Autodesk Inventor part; units mm, degrees
(part 5 of 6)
  line L1795 (9.94, -14.5874) -> (9.724, -14.8873) construction
  line L1796 (9.724, -14.8873) -> (9.508, -15.1933) construction
  line L1797 (9.508, -15.1933) -> (9.2861, -15.4933) construction
  line L1798 (9.2861, -15.4933) -> (8.986, -15.8833)
  line L1799 (8.986, -15.8833) -> (8.8241, -16.0813)
  spline S547 degree 3 poles (8.8241, -16.0813) (8.8061, -16.1053) (8.6861, -16.2073) (8.6921, -16.2433) knots 58 58 58 58 59 59 59 59
  line L1800 (8.8241, -16.0813) -> (8.8061, -16.1053) construction
  line L1801 (8.8061, -16.1053) -> (8.6861, -16.2073) construction
  line L1802 (8.6861, -16.2073) -> (8.6921, -16.2433) construction
  spline S548 degree 3 poles (8.6921, -16.2433) (8.6981, -16.2553) (8.794, -16.1713) (8.8, -16.1653) knots 59 59 59 59 60 60 60 60
  line L1803 (8.6921, -16.2433) -> (8.6981, -16.2553) construction
  line L1804 (8.6981, -16.2553) -> (8.794, -16.1713) construction
  line L1805 (8.794, -16.1713) -> (8.8, -16.1653) construction
  spline S549 degree 3 poles (8.8, -16.1653) (8.728, -16.2433) (8.6321, -16.3513) (8.524, -16.3753) knots 60 60 60 60 61 61 61 61
  line L1806 (8.8, -16.1653) -> (8.728, -16.2433) construction
  line L1807 (8.728, -16.2433) -> (8.6321, -16.3513) construction
  line L1808 (8.6321, -16.3513) -> (8.524, -16.3753) construction
  spline S550 degree 3 poles (8.524, -16.3753) (8.4821, -16.3333) (8.4821, -16.2673) (8.4821, -16.2073) (8.4821, -15.9613) (8.5721, -15.7033) (8.6381, -15.4693) knots 61 61 61 61 62 62 62 63 63 63 63
  line L1809 (8.524, -16.3753) -> (8.4821, -16.3333) construction
  line L1810 (8.4821, -16.3333) -> (8.4821, -16.2673) construction
  line L1811 (8.4821, -16.2673) -> (8.4821, -16.2073) construction
  line L1812 (8.4821, -16.2073) -> (8.4821, -15.9613) construction
  line L1813 (8.4821, -15.9613) -> (8.5721, -15.7033) construction
  line L1814 (8.5721, -15.7033) -> (8.6381, -15.4693) construction
  spline S551 degree 3 poles (8.6381, -15.4693) (8.788, -14.9773) (8.932, -14.4854) (9.112, -14.0054) knots 63 63 63 63 64 64 64 64
  line L1815 (8.6381, -15.4693) -> (8.788, -14.9773) construction
  line L1816 (8.788, -14.9773) -> (8.932, -14.4854) construction
  line L1817 (8.932, -14.4854) -> (9.112, -14.0054) construction
  spline S552 degree 3 poles (9.112, -14.0054) (9.202, -13.7594) (9.304, -13.5194) (9.406, -13.2854) knots 64 64 64 64 65 65 65 65
  line L1818 (9.112, -14.0054) -> (9.202, -13.7594) construction
  line L1819 (9.202, -13.7594) -> (9.304, -13.5194) construction
  line L1820 (9.304, -13.5194) -> (9.406, -13.2854) construction
  spline S553 degree 3 poles (9.406, -13.2854) (9.454, -13.1654) (9.508, -13.0454) (9.562, -12.9254) knots 65 65 65 65 66 66 66 66
  line L1821 (9.406, -13.2854) -> (9.454, -13.1654) construction
  line L1822 (9.454, -13.1654) -> (9.508, -13.0454) construction
  line L1823 (9.508, -13.0454) -> (9.562, -12.9254) construction
  spline S554 degree 3 poles (9.562, -12.9254) (9.604, -12.8414) (9.664, -12.6314) (9.748, -12.6014) knots 66 66 66 66 67 67 67 67
  line L1824 (9.562, -12.9254) -> (9.604, -12.8414) construction
  line L1825 (9.604, -12.8414) -> (9.664, -12.6314) construction
  line L1826 (9.664, -12.6314) -> (9.748, -12.6014) construction
  spline S555 degree 3 poles (9.748, -12.6014) (9.784, -12.5834) (9.844, -12.5954) (9.886, -12.5834) knots 67 67 67 67 68 68 68 68
  line L1827 (9.748, -12.6014) -> (9.784, -12.5834) construction
  line L1828 (9.784, -12.5834) -> (9.844, -12.5954) construction
  line L1829 (9.844, -12.5954) -> (9.886, -12.5834) construction
  spline S556 degree 3 poles (9.886, -12.5834) (9.916, -12.5714) (9.904, -12.5534) (9.934, -12.5474) knots 68 68 68 68 69 69 69 69
  line L1830 (9.886, -12.5834) -> (9.916, -12.5714) construction
  line L1831 (9.916, -12.5714) -> (9.904, -12.5534) construction
  line L1832 (9.904, -12.5534) -> (9.934, -12.5474) construction
  spline S557 degree 3 poles (9.934, -12.5474) (10.006, -12.5354) (10.12, -12.5714) (10.192, -12.5654) knots 69 69 69 69 70 70 70 70
  line L1833 (9.934, -12.5474) -> (10.006, -12.5354) construction
  line L1834 (10.006, -12.5354) -> (10.12, -12.5714) construction
  line L1835 (10.12, -12.5714) -> (10.192, -12.5654) construction
  spline S558 degree 3 poles (10.192, -12.5654) (10.288, -12.5654) (10.624, -12.5174) (10.576, -12.3554) knots 70 70 70 70 71 71 71 71
  line L1836 (10.192, -12.5654) -> (10.288, -12.5654) construction
  line L1837 (10.288, -12.5654) -> (10.624, -12.5174) construction
  line L1838 (10.624, -12.5174) -> (10.576, -12.3554) construction
  spline S559 degree 3 poles (10.576, -12.3554) (10.564, -12.3134) (10.546, -12.3254) (10.516, -12.3254) knots 71 71 71 71 72 72 72 72
  line L1839 (10.576, -12.3554) -> (10.564, -12.3134) construction
  line L1840 (10.564, -12.3134) -> (10.546, -12.3254) construction
  line L1841 (10.546, -12.3254) -> (10.516, -12.3254) construction
  spline S560 degree 3 poles (10.516, -12.3254) (10.492, -12.3194) (10.51, -12.3494) (10.504, -12.3494) knots 72 72 72 72 73 73 73 73
  line L1842 (10.516, -12.3254) -> (10.492, -12.3194) construction
  line L1843 (10.492, -12.3194) -> (10.51, -12.3494) construction
  line L1844 (10.51, -12.3494) -> (10.504, -12.3494) construction
  spline S561 degree 3 poles (10.504, -12.3494) (10.474, -12.3554) (10.438, -12.3554) (10.402, -12.3554) knots 73 73 73 73 74 74 74 74
  line L1845 (10.504, -12.3494) -> (10.474, -12.3554) construction
  line L1846 (10.474, -12.3554) -> (10.438, -12.3554) construction
  line L1847 (10.438, -12.3554) -> (10.402, -12.3554) construction
  line L1848 (10.402, -12.3554) -> (9.826, -12.3794)
  spline S562 degree 3 poles (9.826, -12.3794) (9.826, -12.3794) (9.826, -12.3614) (9.838, -12.3434) knots 75 75 75 75 76 76 76 76
  line L1849 (9.826, -12.3794) -> (9.826, -12.3794) construction
  line L1850 (9.826, -12.3794) -> (9.826, -12.3614) construction
  line L1851 (9.826, -12.3614) -> (9.838, -12.3434) construction
  spline S563 degree 3 poles (9.838, -12.3434) (9.82, -12.3674) (9.808, -12.3794) (9.796, -12.3794) knots 76 76 76 76 77 77 77 77
  line L1852 (9.838, -12.3434) -> (9.82, -12.3674) construction
  line L1853 (9.82, -12.3674) -> (9.808, -12.3794) construction
  line L1854 (9.808, -12.3794) -> (9.796, -12.3794) construction
  spline S564 degree 3 poles (9.796, -12.3794) (9.958, -12.0554) (10.126, -11.7254) (10.33, -11.4194) knots 77 77 77 77 78 78 78 78
  line L1855 (9.796, -12.3794) -> (9.958, -12.0554) construction
  line L1856 (9.958, -12.0554) -> (10.126, -11.7254) construction
  line L1857 (10.126, -11.7254) -> (10.33, -11.4194) construction
  spline S565 degree 3 poles (10.33, -11.4194) (10.324, -11.4314) (10.234, -11.5874) (10.24, -11.5874) knots 78 78 78 78 79 79 79 79
  line L1858 (10.33, -11.4194) -> (10.324, -11.4314) construction
  line L1859 (10.324, -11.4314) -> (10.234, -11.5874) construction
  line L1860 (10.234, -11.5874) -> (10.24, -11.5874) construction
  spline S566 degree 3 poles (10.24, -11.5874) (10.258, -11.5934) (10.492, -11.2574) (10.492, -11.2214) (10.492, -11.2094) (10.468, -11.2334) (10.45, -11.2514) knots 79 79 79 79 80 80 80 81 81 81 81
  line L1861 (10.24, -11.5874) -> (10.258, -11.5934) construction
  line L1862 (10.258, -11.5934) -> (10.492, -11.2574) construction
  line L1863 (10.492, -11.2574) -> (10.492, -11.2214) construction
  line L1864 (10.492, -11.2214) -> (10.492, -11.2094) construction
  line L1865 (10.492, -11.2094) -> (10.468, -11.2334) construction
  line L1866 (10.468, -11.2334) -> (10.45, -11.2514) construction
  spline S567 degree 3 poles (10.45, -11.2514) (10.522, -11.1614) (10.63, -11.0714) (10.48, -10.9814) knots 81 81 81 81 82 82 82 82
  line L1867 (10.45, -11.2514) -> (10.522, -11.1614) construction
  line L1868 (10.522, -11.1614) -> (10.63, -11.0714) construction
  line L1869 (10.63, -11.0714) -> (10.48, -10.9814) construction
  spline S568 degree 3 poles (10.48, -10.9814) (10.348, -10.9034) (10.102, -10.9214) (9.97, -10.9934) knots 82 82 82 82 83 83 83 83
  line L1870 (10.48, -10.9814) -> (10.348, -10.9034) construction
  line L1871 (10.348, -10.9034) -> (10.102, -10.9214) construction
  line L1872 (10.102, -10.9214) -> (9.97, -10.9934) construction
  spline S569 degree 3 poles (9.97, -10.9934) (9.862, -11.0474) (9.808, -11.1674) (9.748, -11.2634) knots 83 83 83 83 84 84 84 84
  line L1873 (9.97, -10.9934) -> (9.862, -11.0474) construction
  line L1874 (9.862, -11.0474) -> (9.808, -11.1674) construction
  line L1875 (9.808, -11.1674) -> (9.748, -11.2634) construction
  spline S570 degree 3 poles (9.748, -11.2634) (9.67, -11.3834) (9.616, -11.4974) (9.562, -11.6234) knots 84 84 84 84 85 85 85 85
  line L1876 (9.748, -11.2634) -> (9.67, -11.3834) construction
  line L1877 (9.67, -11.3834) -> (9.616, -11.4974) construction
  line L1878 (9.616, -11.4974) -> (9.562, -11.6234) construction
  spline S571 degree 3 poles (9.562, -11.6234) (9.538, -11.6774) (9.502, -11.6954) (9.472, -11.7374) knots 85 85 85 85 86 86 86 86
  line L1879 (9.562, -11.6234) -> (9.538, -11.6774) construction
  line L1880 (9.538, -11.6774) -> (9.502, -11.6954) construction
  line L1881 (9.502, -11.6954) -> (9.472, -11.7374) construction
  spline S572 degree 3 poles (9.472, -11.7374) (9.406, -11.8214) (9.364, -11.9174) (9.316, -12.0074) knots 86 86 86 86 87 87 87 87
  line L1882 (9.472, -11.7374) -> (9.406, -11.8214) construction
  line L1883 (9.406, -11.8214) -> (9.364, -11.9174) construction
  line L1884 (9.364, -11.9174) -> (9.316, -12.0074) construction
  line L1885 (9.316, -12.0074) -> (9.19, -12.2894)
  spline S573 degree 3 poles (9.19, -12.2894) (9.13, -12.4274) (9.142, -12.4154) (9.004, -12.4154) knots 88 88 88 88 89 89 89 89
  line L1886 (9.19, -12.2894) -> (9.13, -12.4274) construction
  line L1887 (9.13, -12.4274) -> (9.142, -12.4154) construction
  line L1888 (9.142, -12.4154) -> (9.004, -12.4154) construction
  spline S574 degree 3 poles (9.004, -12.4154) (8.788, -12.4214) (8.5721, -12.4274) (8.3561, -12.4274) knots 89 89 89 89 90 90 90 90
  line L1889 (9.004, -12.4154) -> (8.788, -12.4214) construction
  line L1890 (8.788, -12.4214) -> (8.5721, -12.4274) construction
  line L1891 (8.5721, -12.4274) -> (8.3561, -12.4274) construction
  spline S575 degree 3 poles (8.3561, -12.4274) (8.4041, -12.3374) (8.866, -11.3534) (8.914, -11.3114) knots 90 90 90 90 91 91 91 91
  line L1892 (8.3561, -12.4274) -> (8.4041, -12.3374) construction
  line L1893 (8.4041, -12.3374) -> (8.866, -11.3534) construction
  line L1894 (8.866, -11.3534) -> (8.914, -11.3114) construction
  spline S576 degree 3 poles (8.914, -11.3114) (8.872, -11.3354) (8.6861, -11.7014) (8.5361, -12.0074) knots 91 91 91 91 92 92 92 92
  line L1895 (8.914, -11.3114) -> (8.872, -11.3354) construction
  line L1896 (8.872, -11.3354) -> (8.6861, -11.7014) construction
  line L1897 (8.6861, -11.7014) -> (8.5361, -12.0074) construction
  spline S577 degree 3 poles (8.5361, -12.0074) (8.7401, -11.5814) (8.9681, -11.1614) (9.232, -10.7654) knots 92 92 92 92 93 93 93 93
  line L1898 (8.5361, -12.0074) -> (8.7401, -11.5814) construction
  line L1899 (8.7401, -11.5814) -> (8.9681, -11.1614) construction
  line L1900 (8.9681, -11.1614) -> (9.232, -10.7654) construction
  spline S578 degree 3 poles (9.232, -10.7654) (9.226, -10.7774) (9.136, -10.9274) (9.142, -10.9274) knots 93 93 93 93 94 94 94 94
  line L1901 (9.232, -10.7654) -> (9.226, -10.7774) construction
  line L1902 (9.226, -10.7774) -> (9.136, -10.9274) construction
  line L1903 (9.136, -10.9274) -> (9.142, -10.9274) construction
  spline S579 degree 3 poles (9.142, -10.9274) (9.166, -10.9334) (9.388, -10.6154) (9.388, -10.5794) (9.388, -10.5674) (9.37, -10.5854) (9.3521, -10.5974) knots 94 94 94 94 95 95 95 96 96 96 96
  line L1904 (9.142, -10.9274) -> (9.166, -10.9334) construction
  line L1905 (9.166, -10.9334) -> (9.388, -10.6154) construction
  line L1906 (9.388, -10.6154) -> (9.388, -10.5794) construction
  line L1907 (9.388, -10.5794) -> (9.388, -10.5674) construction
  line L1908 (9.388, -10.5674) -> (9.37, -10.5854) construction
  line L1909 (9.37, -10.5854) -> (9.3521, -10.5974) construction
  spline S580 degree 3 poles (9.3521, -10.5974) (9.394, -10.5554) (9.46, -10.5194) (9.46, -10.4534) knots 96 96 96 96 97 97 97 97
  line L1910 (9.3521, -10.5974) -> (9.394, -10.5554) construction
  line L1911 (9.394, -10.5554) -> (9.46, -10.5194) construction
  line L1912 (9.46, -10.5194) -> (9.46, -10.4534) construction
  spline S581 degree 3 poles (9.46, -10.4534) (9.454, -10.3154) (9.256, -10.2974) (9.16, -10.2974) knots 97 97 97 97 98 98 98 98
  line L1913 (9.46, -10.4534) -> (9.454, -10.3154) construction
  line L1914 (9.454, -10.3154) -> (9.256, -10.2974) construction
  line L1915 (9.256, -10.2974) -> (9.16, -10.2974) construction
  spline S582 degree 3 poles (9.16, -10.2974) (9.034, -10.2914) (8.8781, -10.3154) (8.788, -10.4114) knots 98 98 98 98 99 99 99 99
  line L1916 (9.16, -10.2974) -> (9.034, -10.2914) construction
  line L1917 (9.034, -10.2914) -> (8.8781, -10.3154) construction
  line L1918 (8.8781, -10.3154) -> (8.788, -10.4114) construction
  spline S583 degree 3 poles (8.788, -10.4114) (8.716, -10.4894) (8.656, -10.5974) (8.6021, -10.6814) knots 99 99 99 99 100 100 100 100
  line L1919 (8.788, -10.4114) -> (8.716, -10.4894) construction
  line L1920 (8.716, -10.4894) -> (8.656, -10.5974) construction
  line L1921 (8.656, -10.5974) -> (8.6021, -10.6814) construction
  spline S584 degree 3 poles (8.6021, -10.6814) (8.5421, -10.7774) (8.5061, -10.8974) (8.4461, -10.9874) knots 100 100 100 100 101 101 101 101
  line L1922 (8.6021, -10.6814) -> (8.5421, -10.7774) construction
  line L1923 (8.5421, -10.7774) -> (8.5061, -10.8974) construction
  line L1924 (8.5061, -10.8974) -> (8.4461, -10.9874) construction
  spline S585 degree 3 poles (8.4461, -10.9874) (8.392, -11.0594) (8.3201, -11.1314) (8.2661, -11.2274) knots 101 101 101 101 102 102 102 102
  line L1925 (8.4461, -10.9874) -> (8.392, -11.0594) construction
  line L1926 (8.392, -11.0594) -> (8.3201, -11.1314) construction
  line L1927 (8.3201, -11.1314) -> (8.2661, -11.2274) construction
  spline S586 degree 3 poles (8.2661, -11.2274) (8.1341, -11.4794) (8.0261, -11.7374) (7.9061, -11.9954) knots 102 102 102 102 103 103 103 103
  line L1928 (8.2661, -11.2274) -> (8.1341, -11.4794) construction
  line L1929 (8.1341, -11.4794) -> (8.0261, -11.7374) construction
  line L1930 (8.0261, -11.7374) -> (7.9061, -11.9954) construction
  spline S587 degree 3 poles (7.9061, -11.9954) (7.8461, -12.1094) (7.7921, -12.2294) (7.7441, -12.3554) knots 103 103 103 103 104 104 104 104
  line L1931 (7.9061, -11.9954) -> (7.8461, -12.1094) construction
  line L1932 (7.8461, -12.1094) -> (7.7921, -12.2294) construction
  line L1933 (7.7921, -12.2294) -> (7.7441, -12.3554) construction
  line L1934 (7.7441, -12.3554) -> (7.7141, -12.4334)
  spline S588 degree 3 poles (7.7141, -12.4334) (7.6601, -12.5114) (7.7081, -12.4634) (7.6421, -12.4814) knots 105 105 105 105 106 106 106 106
  line L1935 (7.7141, -12.4334) -> (7.6601, -12.5114) construction
  line L1936 (7.6601, -12.5114) -> (7.7081, -12.4634) construction
  line L1937 (7.7081, -12.4634) -> (7.6421, -12.4814) construction
  spline S589 degree 3 poles (7.6421, -12.4814) (7.5761, -12.4994) (7.4741, -12.4754) (7.4021, -12.4814) knots 106 106 106 106 107 107 107 107
  line L1938 (7.6421, -12.4814) -> (7.5761, -12.4994) construction
  line L1939 (7.5761, -12.4994) -> (7.4741, -12.4754) construction
  line L1940 (7.4741, -12.4754) -> (7.4021, -12.4814) construction
  spline S590 degree 3 poles (7.4021, -12.4814) (7.2375, -12.4849) (7.0587, -12.4887) (6.8833, -12.5042) knots 107 107 107 107 108 108 108 108
  line L1941 (7.4021, -12.4814) -> (7.2375, -12.4849) construction
  line L1942 (7.2375, -12.4849) -> (7.0587, -12.4887) construction
  line L1943 (7.0587, -12.4887) -> (6.8833, -12.5042) construction
  spline S591 degree 3 poles (6.8833, -12.5042) (6.8579, -12.4335) (6.8, -12.348) (6.7361, -12.3074) knots 108 108 108 108 109 109 109 109
  line L1944 (6.8833, -12.5042) -> (6.8579, -12.4335) construction
  line L1945 (6.8579, -12.4335) -> (6.8, -12.348) construction
  line L1946 (6.8, -12.348) -> (6.7361, -12.3074) construction
  spline S592 degree 3 poles (6.7361, -12.3074) (6.6581, -12.2654) (6.5501, -12.2474) (6.4661, -12.2834) knots 109 109 109 109 110 110 110 110
  line L1947 (6.7361, -12.3074) -> (6.6581, -12.2654) construction
  line L1948 (6.6581, -12.2654) -> (6.5501, -12.2474) construction
  line L1949 (6.5501, -12.2474) -> (6.4661, -12.2834) construction
  spline S593 degree 3 poles (6.4661, -12.2834) (6.4481, -12.2894) (6.3761, -12.3074) (6.4001, -12.3314) knots 110 110 110 110 111 111 111 111
  line L1950 (6.4661, -12.2834) -> (6.4481, -12.2894) construction
  line L1951 (6.4481, -12.2894) -> (6.3761, -12.3074) construction
  line L1952 (6.3761, -12.3074) -> (6.4001, -12.3314) construction
  spline S594 degree 3 poles (6.4001, -12.3314) (6.4061, -12.3434) (6.4121, -12.3434) (6.4241, -12.3434) knots 111 111 111 111 112 112 112 112
  line L1953 (6.4001, -12.3314) -> (6.4061, -12.3434) construction
  line L1954 (6.4061, -12.3434) -> (6.4121, -12.3434) construction
  line L1955 (6.4121, -12.3434) -> (6.4241, -12.3434) construction
  spline S595 degree 3 poles (6.4241, -12.3434) (6.3701, -12.3854) (6.2801, -12.4574) (6.4061, -12.5054) knots 112 112 112 112 113 113 113 113
  line L1956 (6.4241, -12.3434) -> (6.3701, -12.3854) construction
  line L1957 (6.3701, -12.3854) -> (6.2801, -12.4574) construction
  line L1958 (6.2801, -12.4574) -> (6.4061, -12.5054) construction
  spline S596 degree 3 poles (6.4061, -12.5054) (6.3941, -12.5174) (6.4061, -12.5714) (6.4061, -12.5774) knots 113 113 113 113 114 114 114 114
  line L1959 (6.4061, -12.5054) -> (6.3941, -12.5174) construction
  line L1960 (6.3941, -12.5174) -> (6.4061, -12.5714) construction
  line L1961 (6.4061, -12.5714) -> (6.4061, -12.5774) construction
  spline S597 degree 3 poles (6.4061, -12.5774) (6.406, -12.5784) (6.4056, -12.58) (6.4053, -12.5812) knots 114 114 114 114 115 115 115 115
  line L1962 (6.4061, -12.5774) -> (6.406, -12.5784) construction
  line L1963 (6.406, -12.5784) -> (6.4056, -12.58) construction
  line L1964 (6.4056, -12.58) -> (6.4053, -12.5812) construction
  spline S598 degree 3 poles (6.4053, -12.5812) (6.3123, -12.6004) (6.1983, -12.6291) (6.2021, -12.6554) knots 115 115 115 115 116 116 116 116
  line L1965 (6.4053, -12.5812) -> (6.3123, -12.6004) construction
  line L1966 (6.3123, -12.6004) -> (6.1983, -12.6291) construction
  line L1967 (6.1983, -12.6291) -> (6.2021, -12.6554) construction
  spline S599 degree 3 poles (6.2021, -12.6554) (6.204, -12.688) (6.2699, -12.7059) (6.361, -12.7151) knots 116 116 116 116 117 117 117 117
  line L1968 (6.2021, -12.6554) -> (6.204, -12.688) construction
  line L1969 (6.204, -12.688) -> (6.2699, -12.7059) construction
  line L1970 (6.2699, -12.7059) -> (6.361, -12.7151) construction
  spline S600 degree 3 poles (6.361, -12.7151) (6.3311, -12.7949) (6.292, -12.8896) (6.2621, -12.9494) knots 117 117 117 117 118 118 118 118
  line L1971 (6.361, -12.7151) -> (6.3311, -12.7949) construction
  line L1972 (6.3311, -12.7949) -> (6.292, -12.8896) construction
  line L1973 (6.292, -12.8896) -> (6.2621, -12.9494) construction
  line L1974 (6.2621, -12.9494) -> (6.3341, -12.8414)
  spline S601 degree 3 poles (6.3341, -12.8414) (6.2921, -12.9314) (6.2441, -13.0154) (6.1901, -13.0874) knots 119 119 119 119 120 120 120 120
  line L1975 (6.3341, -12.8414) -> (6.2921, -12.9314) construction
  line L1976 (6.2921, -12.9314) -> (6.2441, -13.0154) construction
  line L1977 (6.2441, -13.0154) -> (6.1901, -13.0874) construction
  spline S602 degree 3 poles (6.1901, -13.0874) (6.2261, -13.0094) (6.1541, -13.0994) (6.1541, -13.1174) knots 120 120 120 120 121 121 121 121
  line L1978 (6.1901, -13.0874) -> (6.2261, -13.0094) construction
  line L1979 (6.2261, -13.0094) -> (6.1541, -13.0994) construction
  line L1980 (6.1541, -13.0994) -> (6.1541, -13.1174) construction
  spline S603 degree 3 poles (6.1541, -13.1174) (6.0881, -13.0874) (6.1061, -13.2734) (6.1121, -13.2914) knots 121 121 121 121 122 122 122 122
  line L1981 (6.1541, -13.1174) -> (6.0881, -13.0874) construction
  line L1982 (6.0881, -13.0874) -> (6.1061, -13.2734) construction
  line L1983 (6.1061, -13.2734) -> (6.1121, -13.2914) construction
  spline S604 degree 3 poles (6.1121, -13.2914) (6.1121, -13.2974) (6.1481, -13.3513) (6.1481, -13.3514) knots 122 122 122 122 123 123 123 123
  line L1984 (6.1121, -13.2914) -> (6.1121, -13.2974) construction
  line L1985 (6.1121, -13.2974) -> (6.1481, -13.3514) construction
  line L1986 (6.1481, -13.3514) -> (6.1481, -13.3514) construction
  spline S605 degree 3 poles (6.1481, -13.3514) (6.1601, -13.3694) (6.1421, -13.3934) (6.1841, -13.4174) knots 123 123 123 123 124 124 124 124
  line L1987 (6.1481, -13.3514) -> (6.1601, -13.3694) construction
  line L1988 (6.1601, -13.3694) -> (6.1421, -13.3934) construction
  line L1989 (6.1421, -13.3934) -> (6.1841, -13.4174) construction
  spline S606 degree 3 poles (6.1841, -13.4174) (6.2261, -13.4354) (6.2501, -13.4114) (6.2861, -13.3994) knots 124 124 124 124 125 125 125 125
  line L1990 (6.1841, -13.4174) -> (6.2261, -13.4354) construction
  line L1991 (6.2261, -13.4354) -> (6.2501, -13.4114) construction
  line L1992 (6.2501, -13.4114) -> (6.2861, -13.3994) construction
  spline S607 degree 3 poles (6.2861, -13.3994) (6.3581, -13.3694) (6.4121, -13.2914) (6.4661, -13.2434) knots 125 125 125 125 126 126 126 126
  line L1993 (6.2861, -13.3994) -> (6.3581, -13.3694) construction
  line L1994 (6.3581, -13.3694) -> (6.4121, -13.2914) construction
  line L1995 (6.4121, -13.2914) -> (6.4661, -13.2434) construction
  spline S608 degree 3 poles (6.4661, -13.2434) (6.4841, -13.2314) (6.4481, -13.2374) (6.4481, -13.2374) knots 126 126 126 126 127 127 127 127
  line L1996 (6.4661, -13.2434) -> (6.4841, -13.2314) construction
  line L1997 (6.4841, -13.2314) -> (6.4481, -13.2374) construction
  line L1998 (6.4481, -13.2374) -> (6.4481, -13.2374) construction
  spline S609 degree 3 poles (6.4481, -13.2374) (6.5261, -13.1654) (6.4601, -13.2494) (6.5321, -13.2074) knots 127 127 127 127 128 128 128 128
  line L1999 (6.4481, -13.2374) -> (6.5261, -13.1654) construction
  line L2000 (6.5261, -13.1654) -> (6.4601, -13.2494) construction
  line L2001 (6.4601, -13.2494) -> (6.5321, -13.2074) construction
  spline S610 degree 3 poles (6.5321, -13.2074) (6.6041, -13.1594) (6.6161, -13.0814) (6.6761, -13.0154) knots 128 128 128 128 129 129 129 129
  line L2002 (6.5321, -13.2074) -> (6.6041, -13.1594) construction
  line L2003 (6.6041, -13.1594) -> (6.6161, -13.0814) construction
  line L2004 (6.6161, -13.0814) -> (6.6761, -13.0154) construction
  spline S611 degree 3 poles (6.6761, -13.0154) (6.6041, -13.0454) (6.5501, -13.0874) (6.5021, -13.1474) knots 129 129 129 129 130 130 130 130
  line L2005 (6.6761, -13.0154) -> (6.6041, -13.0454) construction
  line L2006 (6.6041, -13.0454) -> (6.5501, -13.0874) construction
  line L2007 (6.5501, -13.0874) -> (6.5021, -13.1474) construction
  spline S612 degree 3 poles (6.5021, -13.1474) (6.4421, -13.2254) (6.4001, -13.2614) (6.3341, -13.3034) knots 130 130 130 130 131 131 131 131
  line L2008 (6.5021, -13.1474) -> (6.4421, -13.2254) construction
  line L2009 (6.4421, -13.2254) -> (6.4001, -13.2614) construction
  line L2010 (6.4001, -13.2614) -> (6.3341, -13.3034) construction
  spline S613 degree 3 poles (6.3341, -13.3034) (6.4061, -13.2494) (6.4421, -13.1954) (6.5021, -13.0994) knots 131 131 131 131 132 132 132 132
  line L2011 (6.3341, -13.3034) -> (6.4061, -13.2494) construction
  line L2012 (6.4061, -13.2494) -> (6.4421, -13.1954) construction
  line L2013 (6.4421, -13.1954) -> (6.5021, -13.0994) construction
  spline S614 degree 3 poles (6.5021, -13.0994) (6.5201, -13.0814) (6.5381, -13.0694) (6.5621, -13.0574) knots 132 132 132 132 133 133 133 133
  line L2014 (6.5021, -13.0994) -> (6.5201, -13.0814) construction
  line L2015 (6.5201, -13.0814) -> (6.5381, -13.0694) construction
  line L2016 (6.5381, -13.0694) -> (6.5621, -13.0574) construction
  spline S615 degree 3 poles (6.5621, -13.0574) (6.5441, -13.0394) (6.5441, -13.0214) (6.5681, -13.0034) knots 133 133 133 133 134 134 134 134
  line L2017 (6.5621, -13.0574) -> (6.5441, -13.0394) construction
  line L2018 (6.5441, -13.0394) -> (6.5441, -13.0214) construction
  line L2019 (6.5441, -13.0214) -> (6.5681, -13.0034) construction
  spline S616 degree 3 poles (6.5681, -13.0034) (6.5861, -12.9734) (6.6221, -12.9614) (6.6401, -12.9314) knots 134 134 134 134 135 135 135 135
  line L2020 (6.5681, -13.0034) -> (6.5861, -12.9734) construction
  line L2021 (6.5861, -12.9734) -> (6.6221, -12.9614) construction
  line L2022 (6.6221, -12.9614) -> (6.6401, -12.9314) construction
  spline S617 degree 3 poles (6.6401, -12.9314) (6.6701, -12.8894) (6.6641, -12.8354) (6.7001, -12.7934) knots 135 135 135 135 136 136 136 136
  line L2023 (6.6401, -12.9314) -> (6.6701, -12.8894) construction
  line L2024 (6.6701, -12.8894) -> (6.6641, -12.8354) construction
  line L2025 (6.6641, -12.8354) -> (6.7001, -12.7934) construction
  spline S618 degree 3 poles (6.7001, -12.7934) (6.7301, -12.7694) (6.7721, -12.7514) (6.7961, -12.7274) knots 136 136 136 136 137 137 137 137
  line L2026 (6.7001, -12.7934) -> (6.7301, -12.7694) construction
  line L2027 (6.7301, -12.7694) -> (6.7721, -12.7514) construction
  line L2028 (6.7721, -12.7514) -> (6.7961, -12.7274) construction
  spline S619 degree 3 poles (6.7961, -12.7274) (6.7989, -12.7249) (6.8017, -12.7219) (6.8045, -12.7192) knots 137 137 137 137 138 138 138 138
  line L2029 (6.7961, -12.7274) -> (6.7989, -12.7249) construction
  line L2030 (6.7989, -12.7249) -> (6.8017, -12.7219) construction
  line L2031 (6.8017, -12.7219) -> (6.8045, -12.7192) construction
  spline S620 degree 3 poles (6.8045, -12.7192) (6.8587, -12.7172) (6.8997, -12.7154) (6.9161, -12.7154) knots 138 138 138 138 139 139 139 139
  line L2032 (6.8045, -12.7192) -> (6.8587, -12.7172) construction
  line L2033 (6.8587, -12.7172) -> (6.8997, -12.7154) construction
  line L2034 (6.8997, -12.7154) -> (6.9161, -12.7154) construction
  spline S621 degree 3 poles (6.9161, -12.7154) (7.0721, -12.7094) (7.2341, -12.7214) (7.3901, -12.7094) knots 139 139 139 139 140 140 140 140
  line L2035 (6.9161, -12.7154) -> (7.0721, -12.7094) construction
  line L2036 (7.0721, -12.7094) -> (7.2341, -12.7214) construction
  line L2037 (7.2341, -12.7214) -> (7.3901, -12.7094) construction
  spline S622 degree 3 poles (7.3901, -12.7094) (7.4741, -12.7034) (7.5461, -12.6734) (7.6241, -12.6674) knots 140 140 140 140 141 141 141 141
  line L2038 (7.3901, -12.7094) -> (7.4741, -12.7034) construction
  line L2039 (7.4741, -12.7034) -> (7.5461, -12.6734) construction
  line L2040 (7.5461, -12.6734) -> (7.6241, -12.6674) construction
  line L2041 (7.6241, -12.6674) -> (7.5401, -12.8834)
  spline S623 degree 3 poles (7.5401, -12.8834) (7.5161, -12.9434) (7.4501, -13.0334) (7.4501, -13.0994) (7.4501, -13.1114) (7.4801, -13.0634) (7.4921, -13.0334) knots 142 142 142 142 143 143 143 144 144 144 144
  line L2042 (7.5401, -12.8834) -> (7.5161, -12.9434) construction
  line L2043 (7.5161, -12.9434) -> (7.4501, -13.0334) construction
  line L2044 (7.4501, -13.0334) -> (7.4501, -13.0994) construction
  line L2045 (7.4501, -13.0994) -> (7.4501, -13.1114) construction
  line L2046 (7.4501, -13.1114) -> (7.4801, -13.0634) construction
  line L2047 (7.4801, -13.0634) -> (7.4921, -13.0334) construction
  line L2048 (7.4921, -13.0334) -> (7.3841, -13.3214)
  spline S624 degree 3 poles (7.3841, -13.3214) (7.3781, -13.3214) (7.4021, -13.2434) (7.3961, -13.2434) knots 145 145 145 145 146 146 146 146
  line L2049 (7.3841, -13.3214) -> (7.3781, -13.3214) construction
  line L2050 (7.3781, -13.3214) -> (7.4021, -13.2434) construction
  line L2051 (7.4021, -13.2434) -> (7.3961, -13.2434) construction
  spline S625 degree 3 poles (7.3961, -13.2434) (7.3601, -13.2434) (7.2221, -13.6394) (7.2101, -13.6634) knots 146 146 146 146 147 147 147 147
  line L2052 (7.3961, -13.2434) -> (7.3601, -13.2434) construction
  line L2053 (7.3601, -13.2434) -> (7.2221, -13.6394) construction
  line L2054 (7.2221, -13.6394) -> (7.2101, -13.6634) construction
  spline S626 degree 3 poles (7.2101, -13.6634) (7.1601, -13.7997) (7.1101, -13.9361) (7.0732, -14.0751) knots 147 147 147 147 148 148 148 148
  line L2055 (7.2101, -13.6634) -> (7.1601, -13.7997) construction
  line L2056 (7.1601, -13.7997) -> (7.1101, -13.9361) construction
  line L2057 (7.1101, -13.9361) -> (7.0732, -14.0751) construction
  spline S627 degree 3 poles (7.0732, -14.0751) (7.0685, -14.0778) (7.0641, -14.0805) (7.0601, -14.0834) knots 148 148 148 148 149 149 149 149
  line L2058 (7.0732, -14.0751) -> (7.0685, -14.0778) construction
  line L2059 (7.0685, -14.0778) -> (7.0641, -14.0805) construction
  line L2060 (7.0641, -14.0805) -> (7.0601, -14.0834) construction
  spline S628 degree 3 poles (7.0601, -14.0834) (7.0061, -14.1194) (6.7061, -14.5154) (6.7301, -14.5453) knots 149 149 149 149 150 150 150 150
  line L2061 (7.0601, -14.0834) -> (7.0061, -14.1194) construction
  line L2062 (7.0061, -14.1194) -> (6.7061, -14.5154) construction
  line L2063 (6.7061, -14.5154) -> (6.7301, -14.5453) construction
  spline S629 degree 3 poles (6.7301, -14.5453) (6.7481, -14.5453) (6.7601, -14.5453) (6.7721, -14.5333) knots 150 150 150 150 151 151 151 151
  line L2064 (6.7301, -14.5453) -> (6.7481, -14.5453) construction
  line L2065 (6.7481, -14.5453) -> (6.7601, -14.5453) construction
  line L2066 (6.7601, -14.5453) -> (6.7721, -14.5333) construction
  spline S630 degree 3 poles (6.7721, -14.5333) (6.6881, -14.6354) (6.5321, -14.7493) (6.4181, -14.8394) knots 151 151 151 151 152 152 152 152
  line L2067 (6.7721, -14.5333) -> (6.6881, -14.6354) construction
  line L2068 (6.6881, -14.6354) -> (6.5321, -14.7493) construction
  line L2069 (6.5321, -14.7493) -> (6.4181, -14.8394) construction
  spline S631 degree 3 poles (6.4181, -14.8394) (6.3521, -14.8934) (6.1901, -15.0433) (6.0941, -14.9953) knots 152 152 152 152 153 153 153 153
  line L2070 (6.4181, -14.8394) -> (6.3521, -14.8934) construction
  line L2071 (6.3521, -14.8934) -> (6.1901, -15.0433) construction
  line L2072 (6.1901, -15.0433) -> (6.0941, -14.9953) construction
  spline S632 degree 3 poles (6.0941, -14.9953) (5.8901, -14.8934) (6.3041, -14.1734) (6.2861, -14.1674) knots 153 153 153 153 154 154 154 154
  line L2073 (6.0941, -14.9953) -> (5.8901, -14.8934) construction
  line L2074 (5.8901, -14.8934) -> (6.3041, -14.1734) construction
  line L2075 (6.3041, -14.1734) -> (6.2861, -14.1674) construction
  spline S633 degree 3 poles (6.2861, -14.1674) (6.2681, -14.1614) (6.1181, -14.4974) (6.0881, -14.5754) knots 154 154 154 154 155 155 155 155
  line L2076 (6.2861, -14.1674) -> (6.2681, -14.1614) construction
  line L2077 (6.2681, -14.1614) -> (6.1181, -14.4974) construction
  line L2078 (6.1181, -14.4974) -> (6.0881, -14.5754) construction
  spline S634 degree 3 poles (6.0881, -14.5754) (6.1601, -14.3654) (6.2561, -14.1554) (6.3701, -13.9694) knots 155 155 155 155 156 156 156 156
  line L2079 (6.0881, -14.5754) -> (6.1601, -14.3654) construction
  line L2080 (6.1601, -14.3654) -> (6.2561, -14.1554) construction
  line L2081 (6.2561, -14.1554) -> (6.3701, -13.9694) construction
  spline S635 degree 3 poles (6.3701, -13.9694) (6.3641, -13.9874) (6.3461, -14.0174) (6.3581, -14.0174) knots 156 156 156 156 157 157 157 157
  line L2082 (6.3701, -13.9694) -> (6.3641, -13.9874) construction
  line L2083 (6.3641, -13.9874) -> (6.3461, -14.0174) construction
  line L2084 (6.3461, -14.0174) -> (6.3581, -14.0174) construction
  spline S636 degree 3 poles (6.3581, -14.0174) (6.3701, -14.0234) (6.4601, -13.8974) (6.4421, -13.8854) knots 157 157 157 157 158 158 158 158
  line L2085 (6.3581, -14.0174) -> (6.3701, -14.0234) construction
  line L2086 (6.3701, -14.0234) -> (6.4601, -13.8974) construction
  line L2087 (6.4601, -13.8974) -> (6.4421, -13.8854) construction
  spline S637 degree 3 poles (6.4421, -13.8854) (6.4361, -13.8854) (6.4241, -13.8854) (6.4181, -13.8914) knots 158 158 158 158 159 159 159 159
  line L2088 (6.4421, -13.8854) -> (6.4361, -13.8854) construction
  line L2089 (6.4361, -13.8854) -> (6.4241, -13.8854) construction
  line L2090 (6.4241, -13.8854) -> (6.4181, -13.8914) construction
  spline S638 degree 3 poles (6.4181, -13.8914) (6.4361, -13.8734) (6.4661, -13.8674) (6.4661, -13.8314) (6.4661, -13.7714) (6.3281, -13.7114) (6.2801, -13.6934) knots 159 159 159 159 160 160 160 161 161 161 161
  line L2091 (6.4181, -13.8914) -> (6.4361, -13.8734) construction
  line L2092 (6.4361, -13.8734) -> (6.4661, -13.8674) construction
  line L2093 (6.4661, -13.8674) -> (6.4661, -13.8314) construction
  line L2094 (6.4661, -13.8314) -> (6.4661, -13.7714) construction
  line L2095 (6.4661, -13.7714) -> (6.3281, -13.7114) construction
  line L2096 (6.3281, -13.7114) -> (6.2801, -13.6934) construction
  spline S639 degree 3 poles (6.2801, -13.6934) (6.1661, -13.6454) (6.0521, -13.6334) (5.9621, -13.6934) knots 161 161 161 161 162 162 162 162
  line L2097 (6.2801, -13.6934) -> (6.1661, -13.6454) construction
  line L2098 (6.1661, -13.6454) -> (6.0521, -13.6334) construction
  line L2099 (6.0521, -13.6334) -> (5.9621, -13.6934) construction
  spline S640 degree 3 poles (5.9621, -13.6934) (5.8421, -13.7654) (5.8181, -13.9094) (5.7701, -14.0354) knots 162 162 162 162 163 163 163 163
  line L2100 (5.9621, -13.6934) -> (5.8421, -13.7654) construction
  line L2101 (5.8421, -13.7654) -> (5.8181, -13.9094) construction
  line L2102 (5.8181, -13.9094) -> (5.7701, -14.0354) construction
  spline S641 degree 3 poles (5.7701, -14.0354) (5.7581, -14.0714) (5.6441, -14.4974) (5.6681, -14.5034) knots 163 163 163 163 164 164 164 164
  line L2103 (5.7701, -14.0354) -> (5.7581, -14.0714) construction
  line L2104 (5.7581, -14.0714) -> (5.6441, -14.4974) construction
  line L2105 (5.6441, -14.4974) -> (5.6681, -14.5034) construction
  spline S642 degree 3 poles (5.6681, -14.5034) (5.6801, -14.4974) (5.6801, -14.4914) (5.6861, -14.4793) knots 164 164 164 164 165 165 165 165
  line L2106 (5.6681, -14.5034) -> (5.6801, -14.4974) construction
  line L2107 (5.6801, -14.4974) -> (5.6801, -14.4914) construction
  line L2108 (5.6801, -14.4914) -> (5.6861, -14.4793) construction
  line L2109 (5.6861, -14.4793) -> (5.6681, -14.5874)
  spline S643 degree 3 poles (5.6681, -14.5874) (5.6621, -14.5874) (5.6741, -14.5574) (5.6621, -14.5574) (5.6141, -14.5574) (5.6261, -14.7734) (5.6321, -14.8033) knots 166 166 166 166 167 167 167 168 168 168 168
  line L2110 (5.6681, -14.5874) -> (5.6621, -14.5874) construction
  line L2111 (5.6621, -14.5874) -> (5.6741, -14.5574) construction
  line L2112 (5.6741, -14.5574) -> (5.6621, -14.5574) construction
  line L2113 (5.6621, -14.5574) -> (5.6141, -14.5574) construction
  line L2114 (5.6141, -14.5574) -> (5.6261, -14.7734) construction
  line L2115 (5.6261, -14.7734) -> (5.6321, -14.8033) construction
  spline S644 degree 3 poles (5.6321, -14.8033) (5.6561, -14.9113) (5.7401, -14.9893) (5.8061, -15.0793) knots 168 168 168 168 169 169 169 169
  line L2116 (5.6321, -14.8033) -> (5.6561, -14.9113) construction
  line L2117 (5.6561, -14.9113) -> (5.7401, -14.9893) construction
  line L2118 (5.7401, -14.9893) -> (5.8061, -15.0793) construction
  spline S645 degree 3 poles (5.8061, -15.0793) (5.8421, -15.1333) (5.8781, -15.1887) (5.9321, -15.2247) knots 169 169 169 169 170 170 170 170
  line L2119 (5.8061, -15.0793) -> (5.8421, -15.1333) construction
  line L2120 (5.8421, -15.1333) -> (5.8781, -15.1887) construction
  line L2121 (5.8781, -15.1887) -> (5.9321, -15.2247) construction
  spline S646 degree 3 poles (5.9321, -15.2247) (6.0041, -15.2787) (5.9561, -15.2083) (6.0041, -15.25) knots 170 170 170 170 171 171 171 171
  line L2122 (5.9321, -15.2247) -> (6.0041, -15.2787) construction
  line L2123 (6.0041, -15.2787) -> (5.9561, -15.2083) construction
  line L2124 (5.9561, -15.2083) -> (6.0041, -15.25) construction
  line L2125 (6.0041, -15.25) -> (5.9921, -15.25)
  spline S647 degree 3 poles (5.9921, -15.25) (5.9861, -15.2917) (6.2141, -15.3447) (6.2621, -15.3387) knots 172 172 172 172 173 173 173 173
  line L2126 (5.9921, -15.25) -> (5.9861, -15.2917) construction
  line L2127 (5.9861, -15.2917) -> (6.2141, -15.3447) construction
  line L2128 (6.2141, -15.3447) -> (6.2621, -15.3387) construction
  spline S648 degree 3 poles (6.2621, -15.3387) (6.4721, -15.2907) (6.6221, -15.032) (6.7421, -14.87) knots 173 173 173 173 174 174 174 174
  line L2129 (6.2621, -15.3387) -> (6.4721, -15.2907) construction
  line L2130 (6.4721, -15.2907) -> (6.6221, -15.032) construction
  line L2131 (6.6221, -15.032) -> (6.7421, -14.87) construction
  spline S649 degree 3 poles (6.7421, -14.87) (6.8123, -14.7813) (6.8756, -14.692) (6.9378, -14.6019) knots 174 174 174 174 175 175 175 175
  line L2132 (6.7421, -14.87) -> (6.8123, -14.7813) construction
  line L2133 (6.8123, -14.7813) -> (6.8756, -14.692) construction
  line L2134 (6.8756, -14.692) -> (6.9378, -14.6019) construction
  spline S650 degree 3 poles (6.9378, -14.6019) (6.9227, -14.6532) (6.9075, -14.7043) (6.8921, -14.7555) knots 175 175 175 175 176 176 176 176
  line L2135 (6.9378, -14.6019) -> (6.9227, -14.6532) construction
  line L2136 (6.9227, -14.6532) -> (6.9075, -14.7043) construction
  line L2137 (6.9075, -14.7043) -> (6.8921, -14.7555) construction
  spline S651 degree 3 poles (6.8921, -14.7555) (6.8621, -14.8575) (6.8329, -14.9594) (6.8149, -15.0614) knots 176 176 176 176 177 177 177 177
  line L2138 (6.8921, -14.7555) -> (6.8621, -14.8575) construction
  line L2139 (6.8621, -14.8575) -> (6.8329, -14.9594) construction
  line L2140 (6.8329, -14.9594) -> (6.8149, -15.0614) construction
  spline S652 degree 3 poles (6.8149, -15.0614) (6.8029, -15.1034) (6.7917, -15.1453) (6.7917, -15.1873) (6.7917, -15.1993) (6.7917, -15.2713) (6.7917, -15.2713) knots 177 177 177 177 178 178 178 179 179 179 179
  line L2141 (6.8149, -15.0614) -> (6.8029, -15.1034) construction
  line L2142 (6.8029, -15.1034) -> (6.7917, -15.1453) construction
  line L2143 (6.7917, -15.1453) -> (6.7917, -15.1873) construction
  line L2144 (6.7917, -15.1873) -> (6.7917, -15.1993) construction
  line L2145 (6.7917, -15.1993) -> (6.7917, -15.2713) construction
  line L2146 (6.7917, -15.2713) -> (6.7917, -15.2713) construction
  line L2147 (6.7917, -15.2713) -> (6.7841, -15.3083)
  spline S653 degree 3 poles (6.7841, -15.3083) (6.7849, -15.2996) (6.7845, -15.2923) (6.7845, -15.2893) knots 180 180 180 180 181 181 181 181
  line L2148 (6.7841, -15.3083) -> (6.7849, -15.2996) construction
  line L2149 (6.7849, -15.2996) -> (6.7845, -15.2923) construction
  line L2150 (6.7845, -15.2923) -> (6.7845, -15.2893) construction
  spline S654 degree 3 poles (6.7845, -15.2893) (6.7485, -15.3253) (6.7483, -15.5833) (6.7363, -15.6313) knots 181 181 181 181 182 182 182 182
  line L2151 (6.7845, -15.2893) -> (6.7485, -15.3253) construction
  line L2152 (6.7485, -15.3253) -> (6.7483, -15.5833) construction
  line L2153 (6.7483, -15.5833) -> (6.7363, -15.6313) construction
  spline S655 degree 3 poles (6.7363, -15.6313) (6.7123, -15.7693) (6.7122, -15.8713) (6.8022, -15.9913) knots 182 182 182 182 183 183 183 183
  line L2154 (6.7363, -15.6313) -> (6.7123, -15.7693) construction
  line L2155 (6.7123, -15.7693) -> (6.7122, -15.8713) construction
  line L2156 (6.7122, -15.8713) -> (6.8022, -15.9913) construction
  spline S656 degree 3 poles (6.8022, -15.9913) (6.8982, -16.1173) (7.1201, -16.2673) (7.2881, -16.1953) knots 183 183 183 183 184 184 184 184
  line L2157 (6.8022, -15.9913) -> (6.8982, -16.1173) construction
  line L2158 (6.8982, -16.1173) -> (7.1201, -16.2673) construction
  line L2159 (7.1201, -16.2673) -> (7.2881, -16.1953) construction
  spline S657 degree 3 poles (7.2881, -16.1953) (7.3961, -16.1473) (7.4801, -16.0273) (7.5521, -15.9433) knots 184 184 184 184 185 185 185 185
  line L2160 (7.2881, -16.1953) -> (7.3961, -16.1473) construction
  line L2161 (7.3961, -16.1473) -> (7.4801, -16.0273) construction
  line L2162 (7.4801, -16.0273) -> (7.5521, -15.9433) construction
  spline S658 degree 3 poles (7.5521, -15.9433) (7.7921, -15.6433) (7.9961, -15.3133) (8.2001, -14.9833) knots 185 185 185 185 186 186 186 186
  line L2163 (7.5521, -15.9433) -> (7.7921, -15.6433) construction
  line L2164 (7.7921, -15.6433) -> (7.9961, -15.3133) construction
  line L2165 (7.9961, -15.3133) -> (8.2001, -14.9833) construction
  spline S659 degree 3 poles (8.2001, -14.9833) (8.1521, -15.2173) (8.1041, -15.4453) (8.0501, -15.6733) knots 186 186 186 186 187 187 187 187
  line L2166 (8.2001, -14.9833) -> (8.1521, -15.2173) construction
  line L2167 (8.1521, -15.2173) -> (8.1041, -15.4453) construction
  line L2168 (8.1041, -15.4453) -> (8.0501, -15.6733) construction
  spline S660 degree 3 poles (8.0501, -15.6733) (8.0261, -15.7813) (7.9952, -15.8893) (7.9772, -15.9973) knots 187 187 187 187 188 188 188 188
  line L2169 (8.0501, -15.6733) -> (8.0261, -15.7813) construction
  line L2170 (8.0261, -15.7813) -> (7.9952, -15.8893) construction
  line L2171 (7.9952, -15.8893) -> (7.9772, -15.9973) construction
  spline S661 degree 3 poles (7.9772, -15.9973) (7.9712, -16.0333) (7.9583, -16.0693) (7.9583, -16.1113) (7.9583, -16.1173) (7.9583, -16.2132) (7.9583, -16.2133) knots 188 188 188 188 189 189 189 190 190 190 190
  line L2172 (7.9772, -15.9973) -> (7.9712, -16.0333) construction
  line L2173 (7.9712, -16.0333) -> (7.9583, -16.0693) construction
  line L2174 (7.9583, -16.0693) -> (7.9583, -16.1113) construction
  line L2175 (7.9583, -16.1113) -> (7.9583, -16.1173) construction
  line L2176 (7.9583, -16.1173) -> (7.9583, -16.2133) construction
  line L2177 (7.9583, -16.2133) -> (7.9583, -16.2133) construction
  spline S662 degree 3 poles (7.9583, -16.2133) (7.9583, -16.2252) (7.9588, -16.2366) (7.9594, -16.2479) knots 190 190 190 190 191 191 191 191
  line L2178 (7.9583, -16.2133) -> (7.9583, -16.2252) construction
  line L2179 (7.9583, -16.2252) -> (7.9588, -16.2366) construction
  line L2180 (7.9588, -16.2366) -> (7.9594, -16.2479) construction
  spline S663 degree 3 poles (7.9594, -16.2479) (7.9308, -16.2905) (7.9826, -16.4364) (7.9884, -16.4653) knots 191 191 191 191 192 192 192 192
  line L2181 (7.9594, -16.2479) -> (7.9308, -16.2905) construction
  line L2182 (7.9308, -16.2905) -> (7.9826, -16.4364) construction
  line L2183 (7.9826, -16.4364) -> (7.9884, -16.4653) construction
  spline S664 degree 3 poles (7.9884, -16.4653) (8.0244, -16.5673) (8.0912, -16.6693) (8.1812, -16.7353) knots 192 192 192 192 193 193 193 193
  line L2184 (7.9884, -16.4653) -> (8.0244, -16.5673) construction
  line L2185 (8.0244, -16.5673) -> (8.0912, -16.6693) construction
  line L2186 (8.0912, -16.6693) -> (8.1812, -16.7353) construction
  spline S665 degree 3 poles (8.1812, -16.7353) (8.2712, -16.8073) (8.4156, -16.8673) (8.5356, -16.8193) knots 193 193 193 193 194 194 194 194
  line L2187 (8.1812, -16.7353) -> (8.2712, -16.8073) construction
  line L2188 (8.2712, -16.8073) -> (8.4156, -16.8673) construction
  line L2189 (8.4156, -16.8673) -> (8.5356, -16.8193) construction
  spline S666 degree 3 poles (8.5356, -16.8193) (8.7216, -16.7413) (8.8838, -16.4893) (8.9978, -16.3333) knots 194 194 194 194 195 195 195 195
  line L2190 (8.5356, -16.8193) -> (8.7216, -16.7413) construction
  line L2191 (8.7216, -16.7413) -> (8.8838, -16.4893) construction
  line L2192 (8.8838, -16.4893) -> (8.9978, -16.3333) construction
  spline S667 degree 3 poles (8.9978, -16.3333) (9.1898, -16.0873) (9.3639, -15.8233) (9.5439, -15.5653) knots 195 195 195 195 196 196 196 196
  line L2193 (8.9978, -16.3333) -> (9.1898, -16.0873) construction
  line L2194 (9.1898, -16.0873) -> (9.3639, -15.8233) construction
  line L2195 (9.3639, -15.8233) -> (9.5439, -15.5653) construction
  spline S668 degree 3 poles (9.5439, -15.5653) (9.7059, -15.3253) (9.874, -15.0853) (10.024, -14.8334) knots 196 196 196 196 197 197 197 197
  line L2196 (9.5439, -15.5653) -> (9.7059, -15.3253) construction
  line L2197 (9.7059, -15.3253) -> (9.874, -15.0853) construction
  line L2198 (9.874, -15.0853) -> (10.024, -14.8334) construction
  spline S669 degree 3 poles (10.024, -14.8334) (10.072, -14.7554) (10.102, -14.6833) (10.15, -14.6113) knots 197 197 197 197 198 198 198 198
  line L2199 (10.024, -14.8334) -> (10.072, -14.7554) construction
  line L2200 (10.072, -14.7554) -> (10.102, -14.6833) construction
  line L2201 (10.102, -14.6833) -> (10.15, -14.6113) construction
  spline S670 degree 3 poles (10.15, -14.6113) (10.1788, -14.5729) (10.2124, -14.5325) (10.2451, -14.491) knots 198 198 198 198 199 199 199 199
  line L2202 (10.15, -14.6113) -> (10.1788, -14.5729) construction
  line L2203 (10.1788, -14.5729) -> (10.2124, -14.5325) construction
  line L2204 (10.2124, -14.5325) -> (10.2451, -14.491) construction
  spline S671 degree 3 poles (10.2451, -14.491) (10.243, -14.5273) (10.2427, -14.5581) (10.2401, -14.5634) knots 199 199 199 199 200 200 200 200
  line L2205 (10.2451, -14.491) -> (10.243, -14.5273) construction
  line L2206 (10.243, -14.5273) -> (10.2427, -14.5581) construction
  line L2207 (10.2427, -14.5581) -> (10.2401, -14.5634) construction
  spline S672 degree 3 poles (10.2401, -14.5634) (10.1621, -14.8873) (10.0721, -15.2113) (10.0481, -15.5473) knots 200 200 200 200 201 201 201 201
  line L2208 (10.2401, -14.5634) -> (10.1621, -14.8873) construction
  line L2209 (10.1621, -14.8873) -> (10.0721, -15.2113) construction
  line L2210 (10.0721, -15.2113) -> (10.0481, -15.5473) construction
  spline S673 degree 3 poles (10.0481, -15.5473) (10.0301, -15.8653) (10.0301, -16.2853) (10.2821, -16.5193) knots 201 201 201 201 202 202 202 202
  line L2211 (10.0481, -15.5473) -> (10.0301, -15.8653) construction
  line L2212 (10.0301, -15.8653) -> (10.0301, -16.2853) construction
  line L2213 (10.0301, -16.2853) -> (10.2821, -16.5193) construction
  spline S674 degree 3 poles (10.2821, -16.5193) (10.5641, -16.7773) (10.8881, -16.6033) (11.122, -16.3813) knots 202 202 202 202 203 203 203 203
  line L2214 (10.2821, -16.5193) -> (10.5641, -16.7773) construction
  line L2215 (10.5641, -16.7773) -> (10.8881, -16.6033) construction
  line L2216 (10.8881, -16.6033) -> (11.122, -16.3813) construction
  spline S675 degree 3 poles (11.122, -16.3813) (11.3981, -16.1113) (11.632, -15.7933) (11.848, -15.4813) knots 203 203 203 203 204 204 204 204
  line L2217 (11.122, -16.3813) -> (11.3981, -16.1113) construction
  line L2218 (11.3981, -16.1113) -> (11.632, -15.7933) construction
  line L2219 (11.632, -15.7933) -> (11.848, -15.4813) construction
  spline S676 degree 3 poles (11.848, -15.4813) (11.9822, -15.2862) (12.0971, -15.0828) (12.2133, -14.8824) knots 204 204 204 204 205 205 205 205
  line L2220 (11.848, -15.4813) -> (11.9822, -15.2862) construction
  line L2221 (11.9822, -15.2862) -> (12.0971, -15.0828) construction
  line L2222 (12.0971, -15.0828) -> (12.2133, -14.8824) construction
  spline S677 degree 3 poles (12.2133, -14.8824) (12.2056, -14.9297) (12.198, -14.9773) (12.19, -15.0253) knots 205 205 205 205 206 206 206 206
  line L2223 (12.2133, -14.8824) -> (12.2056, -14.9297) construction
  line L2224 (12.2056, -14.9297) -> (12.198, -14.9773) construction
  line L2225 (12.198, -14.9773) -> (12.19, -15.0253) construction
  spline S678 degree 3 poles (12.19, -15.0253) (12.16, -15.2053) (12.142, -15.3733) (12.238, -15.5413) knots 206 206 206 206 207 207 207 207
  line L2226 (12.19, -15.0253) -> (12.16, -15.2053) construction
  line L2227 (12.16, -15.2053) -> (12.142, -15.3733) construction
  line L2228 (12.142, -15.3733) -> (12.238, -15.5413) construction
  spline S679 degree 3 poles (12.238, -15.5413) (12.232, -15.4813) (12.22, -15.4273) (12.22, -15.3733) (12.22, -15.3433) (12.232, -15.3133) (12.232, -15.2893) (12.232, -15.2773) (12.22, -15.2413) (12.22, -15.2233) (12.22, -15.1693) (12.232, -15.1273) (12.244, -15.0733) knots 207 207 207 207 208 208 208 209 209 209 210 210 210 211 211 211 211
  line L2229 (12.238, -15.5413) -> (12.232, -15.4813) construction
  line L2230 (12.232, -15.4813) -> (12.22, -15.4273) construction
  line L2231 (12.22, -15.4273) -> (12.22, -15.3733) construction
  line L2232 (12.22, -15.3733) -> (12.22, -15.3433) construction
  line L2233 (12.22, -15.3433) -> (12.232, -15.3133) construction
  line L2234 (12.232, -15.3133) -> (12.232, -15.2893) construction
  line L2235 (12.232, -15.2893) -> (12.232, -15.2773) construction
  line L2236 (12.232, -15.2773) -> (12.22, -15.2413) construction
  line L2237 (12.22, -15.2413) -> (12.22, -15.2233) construction
  line L2238 (12.22, -15.2233) -> (12.22, -15.1693) construction
  line L2239 (12.22, -15.1693) -> (12.232, -15.1273) construction
  line L2240 (12.232, -15.1273) -> (12.244, -15.0733) construction
  spline S680 degree 3 poles (12.244, -15.0733) (12.25, -15.0193) (12.244, -14.9654) (12.25, -14.9113) knots 211 211 211 211 212 212 212 212
  line L2241 (12.244, -15.0733) -> (12.25, -15.0193) construction
  line L2242 (12.25, -15.0193) -> (12.244, -14.9654) construction
  line L2243 (12.244, -14.9654) -> (12.25, -14.9113) construction
  spline S681 degree 3 poles (12.25, -14.9113) (12.256, -14.8513) (12.28, -14.8033) (12.304, -14.7493) knots 212 212 212 212 213 213 213 213
  line L2244 (12.25, -14.9113) -> (12.256, -14.8513) construction
  line L2245 (12.256, -14.8513) -> (12.28, -14.8033) construction
  line L2246 (12.28, -14.8033) -> (12.304, -14.7493) construction
  spline S682 degree 3 poles (12.304, -14.7493) (12.3101, -14.7332) (12.3146, -14.7179) (12.3188, -14.7027) knots 213 213 213 213 214 214 214 214
  line L2247 (12.304, -14.7493) -> (12.3101, -14.7332) construction
  line L2248 (12.3101, -14.7332) -> (12.3146, -14.7179) construction
  line L2249 (12.3146, -14.7179) -> (12.3188, -14.7027) construction